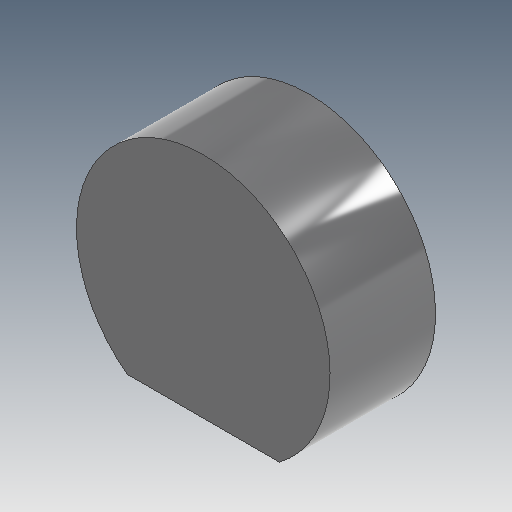
# Autodesk Inventor part: Thermal pad
Saved by Autodesk Inventor 2020.3 (Build 243373010, 373A)
## iProperties
Created: 2021-04-11
Part Number: Thermal pad
Material: Rubber, Silicone
Document SubType Name: Modeling
Designer: marti
Density: 1.25 g/cm^3
Appearance: Silicon Nitride - Polished
Mass: 10.4489 g
Surface Area: 24.996 cm^2
Volume: 8.35913 cm^3
Author: marti
Autodesk Inventor part; units mm, degrees
ref_plane "YZ Plane" through (0, 0, 0) normal (1, 0, 0) x (0, 1, 0)
ref_plane "XZ Plane" through (0, 0, 0) normal (0, 1, 0) x (-1, 0, 0)
ref_plane "XY Plane" through (0, 0, 0) normal (0, 0, 1) x (1, 0, 0)
sketch "Sketch1" plane through (0, 0, 0) normal (0, 0, 1) x (1, 0, 0)
  arc A0 (9, -12) -> (-9, -12) centre (0, 0) ccw
  line L0 (-9, -12) -> (9, -12)
  dimension "d0" = 30
  dimension "d1" = 12
  constraints: 2 end point, 2 point on circle, 1 centre point, 1 coincident, 1 horizontal
  measures "d0" diameter of A0
  measures "d1" distance from line of point (0, 0) L0
extrude "Extrusion1" add sketch "Sketch1" along normal mid plane 12.475
body "Solid1"
